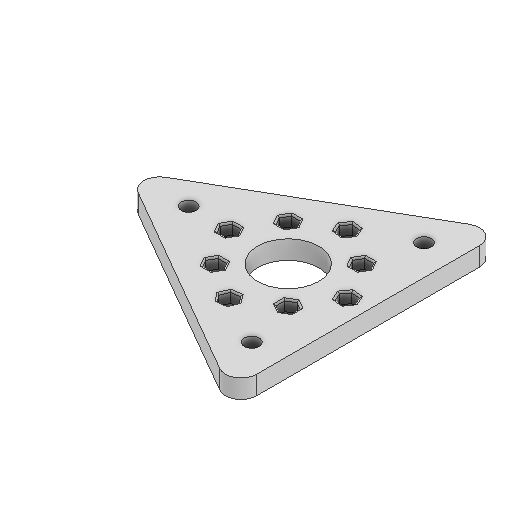
# Autodesk Inventor part: AP-1-02-planetCarrier
Saved by Autodesk Inventor 2025.1 (Build 291241020, 241B)
## iProperties
Created: 2023-07-11
Part Number: AP-1-02-planetCarrier
Material: Generic
Document SubType Name: Modeling
Designer: t205b
Density: 1 g/cm^3
Appearance: Default
Author: t205b
Autodesk Inventor part; units mm, degrees
ref_plane "YZ Plane" through (0, 0, 0) normal (1, 0, 0) x (0, 1, 0)
ref_plane "XZ Plane" through (0, 0, 0) normal (0, 1, 0) x (-1, 0, 0)
ref_plane "XY Plane" through (0, 0, 0) normal (0, 0, 1) x (1, 0, 0)
sketch "Sketch1" plane through (0, 0, 0) normal (0, 1, 0) x (-1, 0, 0)
  line L0 (153.9793, -88.9) -> (0, 0)
  line L1 (0, 0) -> (0, -177.8)
  line L2 (0, -177.8) -> (153.9793, -88.9)
  circle A0 centre (51.3264, -88.9) radius 19.65
  line L3 (76.9897, -133.35) -> (61.1514, -105.9174) construction
  line L4 (76.9897, -44.45) -> (61.1514, -71.8826) construction
  line L5 (31.6764, -88.9) -> (0, -88.9) construction
  circle A1 centre (115.2355, -88.9) radius 6.1085
  circle A2 centre (19.3719, -144.2469) radius 6.1085
  circle A3 centre (19.3719, -33.5531) radius 6.1085
  line L6 (19.3719, -144.2469) -> (51.3264, -88.9) construction
  line L7 (51.3264, -88.9) -> (115.2355, -88.9) construction
  line L8 (51.3264, -88.9) -> (19.3719, -33.5531) construction
  arc A4 (19.8862, -150.3337) -> (18.8576, -150.3337) centre (19.3719, -150.3604) ccw
  arc A5 (21.7419, -149.8769) -> (20.7637, -150.1947) centre (21.2611, -150.0612) ccw
  arc A6 (23.3657, -148.8689) -> (22.5335, -149.4735) centre (22.9653, -149.1928) ccw
  arc A7 (24.5985, -147.4086) -> (23.9939, -148.2407) centre (24.3178, -147.8403) ccw
  arc A8 (25.3197, -145.6387) -> (25.0019, -146.617) centre (25.1862, -146.1361) ccw
  arc A9 (25.4587, -143.7326) -> (25.4587, -144.7612) centre (25.4854, -144.2469) ccw
  arc A10 (25.0019, -141.8768) -> (25.3197, -142.8551) centre (25.1862, -142.3577) ccw
  arc A11 (23.9939, -140.2531) -> (24.5985, -141.0853) centre (24.3178, -140.6535) ccw
  arc A12 (22.5335, -139.0203) -> (23.3657, -139.6249) centre (22.9653, -139.301) ccw
  arc A13 (20.7637, -138.2991) -> (21.7419, -138.6169) centre (21.2611, -138.4326) ccw
  arc A14 (18.8576, -138.1601) -> (19.8862, -138.1601) centre (19.3719, -138.1334) ccw
  arc A15 (17.0018, -138.6169) -> (17.9801, -138.2991) centre (17.4827, -138.4326) ccw
  arc A16 (15.3781, -139.6249) -> (16.2102, -139.0203) centre (15.7785, -139.301) ccw
  arc A17 (14.1452, -141.0853) -> (14.7499, -140.2531) centre (14.426, -140.6535) ccw
  arc A18 (13.4241, -142.8551) -> (13.7419, -141.8768) centre (13.5576, -142.3577) ccw
  arc A19 (13.2851, -144.7612) -> (13.2851, -143.7326) centre (13.2584, -144.2469) ccw
  arc A20 (13.7419, -146.617) -> (13.4241, -145.6387) centre (13.5576, -146.1361) ccw
  arc A21 (14.7499, -148.2407) -> (14.1452, -147.4086) centre (14.426, -147.8403) ccw
  arc A22 (16.2102, -149.4735) -> (15.3781, -148.8689) centre (15.7785, -149.1928) ccw
  arc A23 (17.9801, -150.1947) -> (17.0018, -149.8769) centre (17.4827, -150.0612) ccw
  arc A24 (121.0824, -87.1314) -> (121.2963, -88.1376) centre (121.2155, -87.6289) ccw
  arc A25 (120.2497, -85.4112) -> (120.764, -86.302) centre (120.53, -85.8432) ccw
  arc A26 (118.9262, -84.0325) -> (119.6906, -84.7208) centre (119.3263, -84.3568) ccw
  arc A27 (117.2414, -83.1302) -> (118.1811, -83.5486) centre (117.7221, -83.315) ccw
  arc A28 (115.3603, -82.7928) -> (116.3833, -82.9003) centre (115.8746, -82.82) ccw
  arc A29 (113.467, -83.0531) -> (114.4731, -82.8393) centre (113.9645, -82.9201) ccw
  arc A30 (111.7467, -83.8858) -> (112.6375, -83.3715) centre (112.1788, -83.6056) ccw
  arc A31 (110.368, -85.2093) -> (111.0563, -84.4449) centre (110.6923, -84.8093) ccw
  arc A32 (109.4658, -86.8941) -> (109.8842, -85.9544) centre (109.6506, -86.4134) ccw
  arc A33 (109.1283, -88.7752) -> (109.2358, -87.7523) centre (109.1555, -88.261) ccw
  arc A34 (113.2297, -94.6698) -> (112.29, -94.2514) centre (112.749, -94.485) ccw
  arc A35 (115.1108, -95.0072) -> (114.0878, -94.8997) centre (114.5965, -94.98) ccw
  arc A36 (117.0041, -94.7469) -> (115.998, -94.9607) centre (116.5066, -94.8799) ccw
  arc A37 (118.7244, -93.9142) -> (117.8336, -94.4285) centre (118.2923, -94.1944) ccw
  arc A38 (120.1031, -92.5907) -> (119.4148, -93.3551) centre (119.7788, -92.9907) ccw
  arc A39 (121.0053, -90.9059) -> (120.5869, -91.8456) centre (120.8205, -91.3866) ccw
  arc A40 (121.3428, -89.0248) -> (121.2353, -90.0477) centre (121.3156, -89.539) ccw
  arc A41 (111.5449, -93.7675) -> (110.7805, -93.0792) centre (111.1448, -93.4432) ccw
  arc A42 (110.2214, -92.3888) -> (109.7071, -91.498) centre (109.9411, -91.9567) ccw
  arc A43 (109.3887, -90.6686) -> (109.1748, -89.6624) centre (109.2556, -90.1711) ccw
  arc A44 (14.9168, -29.3738) -> (15.6812, -28.6856) centre (15.2812, -29.0099) ccw
  arc A45 (13.8434, -30.9551) -> (14.3577, -30.0643) centre (14.0774, -30.4963) ccw
  arc A46 (13.3112, -32.7906) -> (13.525, -31.7845) centre (13.392, -32.282) ccw
  arc A47 (13.3722, -34.7008) -> (13.2647, -33.6778) centre (13.2919, -34.1921) ccw
  arc A48 (14.0205, -36.4987) -> (13.6021, -35.559) centre (13.7869, -36.0397) ccw
  arc A49 (15.1926, -38.0082) -> (14.5044, -37.2438) centre (14.8287, -37.6438) ccw
  arc A50 (16.7739, -39.0816) -> (15.8831, -38.5673) centre (16.3151, -38.8475) ccw
  arc A51 (18.6094, -39.6138) -> (17.6033, -39.4) centre (18.1008, -39.533) ccw
  arc A52 (20.5196, -39.5528) -> (19.4966, -39.6603) centre (20.0109, -39.6331) ccw
  arc A53 (22.3175, -38.9045) -> (21.3778, -39.3229) centre (21.8585, -39.138) ccw
  arc A54 (25.3716, -32.4054) -> (25.4791, -33.4283) centre (25.4519, -32.9141) ccw
  arc A55 (24.7233, -30.6075) -> (25.1416, -31.5472) centre (24.9568, -31.0665) ccw
  arc A56 (23.5511, -29.098) -> (24.2394, -29.8624) centre (23.9151, -29.4624) ccw
  arc A57 (21.9699, -28.0246) -> (22.8607, -28.5389) centre (22.4286, -28.2586) ccw
  arc A58 (20.1343, -27.4924) -> (21.1405, -27.7062) centre (20.643, -27.5732) ccw
  arc A59 (18.2241, -27.5534) -> (19.2471, -27.4459) centre (18.7328, -27.4731) ccw
  arc A60 (16.4263, -28.2017) -> (17.366, -27.7833) centre (16.8853, -27.9681) ccw
  arc A61 (25.4326, -34.3155) -> (25.2188, -35.3217) centre (25.3518, -34.8242) ccw
  arc A62 (24.9004, -36.1511) -> (24.3861, -37.0419) centre (24.6663, -36.6098) ccw
  arc A63 (23.827, -37.7323) -> (23.0625, -38.4206) centre (23.4626, -38.0963) ccw
  circle A64 centre (19.3719, -144.2469) radius 4.7879
  circle A65 centre (115.2355, -88.9) radius 4.7879
  circle A66 centre (19.3719, -33.5531) radius 4.7879
  point P0 (21.7419, -149.8769)
  point P1 (23.3657, -148.8689)
  point P2 (22.5335, -149.4735)
  point P3 (24.5985, -147.4086)
  point P4 (25.0019, -141.8768)
  point P5 (25.3197, -142.8551)
  point P6 (23.9939, -140.2531)
  point P7 (22.5335, -139.0203)
  point P8 (23.3657, -139.6249)
  point P9 (20.7637, -138.2991)
  point P10 (21.7419, -138.6169)
  point P11 (19.8862, -138.1601)
  point P12 (17.9801, -138.2991)
  point P13 (15.3781, -139.6249)
  point P14 (16.2102, -139.0203)
  point P15 (14.1452, -141.0853)
  point P16 (14.7499, -140.2531)
  point P17 (13.2851, -144.7612)
  point P18 (13.7419, -146.617)
  point P19 (13.4241, -145.6387)
  point P20 (14.7499, -148.2407)
  point P21 (14.1452, -147.4086)
  point P22 (16.2102, -149.4735)
  point P23 (15.3781, -148.8689)
  point P24 (17.0018, -149.8769)
  point P25 (15.6812, -28.6856)
  point P26 (13.8434, -30.9551)
  point P27 (14.3577, -30.0643)
  point P28 (13.3112, -32.7906)
  point P29 (13.525, -31.7845)
  point P30 (14.0205, -36.4987)
  point P31 (15.1926, -38.0082)
  point P32 (14.5044, -37.2438)
  point P33 (16.7739, -39.0816)
  point P34 (15.8831, -38.5673)
  point P35 (18.6094, -39.6138)
  point P36 (17.6033, -39.4)
  point P37 (20.5196, -39.5528)
  point P38 (19.4966, -39.6603)
  point P39 (22.3175, -38.9045)
  point P40 (21.3778, -39.3229)
  point P41 (25.3716, -32.4054)
  point P42 (25.4791, -33.4283)
  point P43 (24.7233, -30.6075)
  point P44 (25.1416, -31.5472)
  point P45 (23.5511, -29.098)
  point P46 (24.2394, -29.8624)
  point P47 (21.9699, -28.0246)
  point P48 (22.8607, -28.5389)
  point P49 (20.1343, -27.4924)
  point P50 (21.1405, -27.7062)
  point P51 (18.2241, -27.5534)
  point P52 (16.4263, -28.2017)
  point P53 (17.366, -27.7833)
  point P54 (25.2188, -35.3217)
  point P55 (24.9004, -36.1511)
  point P56 (24.3861, -37.0419)
  point P57 (23.827, -37.7323)
  point P58 (23.0625, -38.4206)
  point P59 (121.0824, -87.1314)
  point P60 (120.764, -86.302)
  point P61 (118.1811, -83.5486)
  point P62 (115.3603, -82.7928)
  point P63 (116.3833, -82.9003)
  point P64 (111.7467, -83.8858)
  point P65 (112.6375, -83.3715)
  point P66 (109.8842, -85.9544)
  point P67 (109.2358, -87.7523)
  point P68 (121.3428, -89.0248)
  point P69 (110.2214, -92.3888)
  point P70 (109.7071, -91.498)
  point P71 (109.3887, -90.6686)
  point P72 (109.1748, -89.6624)
  point P73 (113.2297, -94.6698)
  point P74 (112.29, -94.2514)
  point P75 (115.1108, -95.0072)
  point P76 (117.0041, -94.7469)
  point P77 (117.8336, -94.4285)
  point P78 (119.4148, -93.3551)
  dimension "d4" = 12.217
  dimension "d0" = 177.8
  dimension "d1" = 39.3
  dimension "d2" = 102.6529
  dimension "d3" = 63.9091
  dimension "d5" = 120
  dimension "d6" = 120
  dimension "d11" = 0.515
  dimension "d15" = 360
  dimension "d19" = 360
  dimension "d55" = 9.5758
  dimension "d56" = 63.9091
  dimension "d59" = 360
  constraints: 123 point on circle, 64 centre point, 18 end point, 6 equal length, 3 line through centre, 3 midpoint, 2 perpendicular, 1 coincident, 1 horizontal, 1 point on line, 1 vertical, 1 vertical alignment, 337 other
  measures "d0" distance of L0.end L1.end
  measures "d1" diameter of A0
  measures "d2" distance of L1.end L6.end
  measures "d3" distance of L6.start L6.end
  measures "d5" angle of L6 L7
  measures "d6" angle of L8 L7
  measures "d11" radius of A4
  measures "d55" diameter of A64
  measures "d56" distance of A64.centre L6.end
extrude "Extrusion1" add sketch "Sketch1" along normal blind 12 contours L2 L1 L0 | A1 A40 A39 A38 A37 A36 A35 A34 A41 A42 A43 A33 A32 A31 A30 A29 A28 A27 A26 A25 A24 | A24 A1 | A1 A40 | A25 A1 | A1 A39 | A26 A1 | A1 A38 | A27 A1 | A1 A37 | A28 A1 | A1 A36 | A29 A1 | A1 A35 | A30 A1 | A1 A34 | A31 A1 | A1 A41 | A32 A1 | A1 A42 | A33 A1 | A1 A43 | A2 A9 | A9 A2 A8 A7 A6 A5 A4 A23 A22 A21 A20 A19 A18 A17 A16 A15 A14 A13 A12 A11 A10 | A10 A2 | A2 A8 | A11 A2 | A2 A7 | A12 A2 | A2 A6 | A13 A2 | A2 A5 | A14 A2 | A2 A4 | A15 A2 | A2 A23 | A16 A2 | A2 A22 | A17 A2 | A2 A21 | A18 A2 | A2 A20 | A19 A2 | A3 A61 A62 A63 A53 A52 A51 A50 A49 A48 A47 A46 A45 A44 A60 A59 A58 A57 A56 A55 A54 | A54 A3 | A3 A61 | A55 A3 | A3 A62 | A56 A3 | A3 A63 | A57 A3 | A3 A53 | A58 A3 | A3 A52 | A59 A3 | A3 A51 | A60 A3 | A3 A50 | A44 A3 | A3 A49 | A45 A3 | A3 A48 | A46 A3 | A3 A47
fillet "Fillet1" radius 10 3 edges at (0, 6, -177.8) (0, 6, 0) (-153.9793, 6, -88.9)
sketch "Sketch3" plane through (0, 12, 0) normal (0, 1, 0) x (1, 0, 0)
  circle A0 centre (-27.7564, 65.33) radius 2.85
  circle A1 centre (-74.8964, 65.33) radius 2.85
  circle A2 centre (-74.8964, 112.47) radius 2.85
  circle A3 centre (-27.7564, 112.47) radius 2.85
  circle A4 centre (-51.3264, 88.9) radius 19.65 projected
  circle A5 centre (-51.3264, 126.9) radius 2.85
  circle A6 centre (-89.3264, 88.9) radius 2.85
  circle A7 centre (-51.3264, 50.9) radius 2.85
  circle A8 centre (-13.3264, 88.9) radius 2.85
  circle A9 centre (-89.3264, 88.9) radius 5
  circle A10 centre (-51.3264, 50.9) radius 5
  circle A11 centre (-74.8964, 65.33) radius 5
  circle A12 centre (-27.7564, 65.33) radius 5
  circle A13 centre (-13.3264, 88.9) radius 5
  circle A14 centre (-74.8964, 112.47) radius 5
  circle A15 centre (-51.3264, 126.9) radius 5
  circle A16 centre (-27.7564, 112.47) radius 5
  line L0 (-47.8195, 46.3137) -> (-53.5448, 45.5697)
  line L1 (-53.5448, 45.5697) -> (-57.0518, 50.156)
  line L2 (-57.0518, 50.156) -> (-54.8334, 55.4863)
  line L3 (-54.8334, 55.4863) -> (-49.108, 56.2303)
  line L4 (-49.108, 56.2303) -> (-45.6011, 51.644)
  line L5 (-45.6011, 51.644) -> (-47.8195, 46.3137)
  line L6 (-22.7179, 62.511) -> (-27.6785, 59.557)
  line L7 (-27.6785, 59.557) -> (-32.717, 62.376)
  line L8 (-32.717, 62.376) -> (-32.795, 68.149)
  line L9 (-32.795, 68.149) -> (-27.8344, 71.103)
  line L10 (-27.8344, 71.103) -> (-22.7959, 68.284)
  line L11 (-22.7959, 68.284) -> (-22.7179, 62.511)
  line L12 (-10.9778, 83.6258) -> (-16.7197, 84.2289)
  line L13 (-16.7197, 84.2289) -> (-19.0684, 89.5031)
  line L14 (-19.0684, 89.5031) -> (-15.6751, 94.1742)
  line L15 (-15.6751, 94.1742) -> (-9.9332, 93.5711)
  line L16 (-9.9332, 93.5711) -> (-7.5845, 88.2969)
  line L17 (-7.5845, 88.2969) -> (-10.9778, 83.6258)
  line L18 (-21.9829, 112.47) -> (-24.8697, 107.47)
  line L19 (-24.8697, 107.47) -> (-30.6432, 107.47)
  line L20 (-30.6432, 107.47) -> (-33.5299, 112.47)
  line L21 (-33.5299, 112.47) -> (-30.6432, 117.47)
  line L22 (-30.6432, 117.47) -> (-24.8697, 117.47)
  line L23 (-24.8697, 117.47) -> (-21.9829, 112.47)
  line L24 (-45.6011, 126.156) -> (-49.108, 121.5697)
  line L25 (-49.108, 121.5697) -> (-54.8334, 122.3137)
  line L26 (-54.8334, 122.3137) -> (-57.0518, 127.644)
  line L27 (-57.0518, 127.644) -> (-53.5448, 132.2303)
  line L28 (-53.5448, 132.2303) -> (-47.8195, 131.4863)
  line L29 (-47.8195, 131.4863) -> (-45.6011, 126.156)
  line L30 (-72.0097, 107.47) -> (-77.7832, 107.47)
  line L31 (-77.7832, 107.47) -> (-80.6699, 112.47)
  line L32 (-80.6699, 112.47) -> (-77.7832, 117.47)
  line L33 (-77.7832, 117.47) -> (-72.0097, 117.47)
  line L34 (-72.0097, 117.47) -> (-69.1229, 112.47)
  line L35 (-69.1229, 112.47) -> (-72.0097, 107.47)
  line L36 (-83.5529, 88.9) -> (-86.4397, 83.9)
  line L37 (-86.4397, 83.9) -> (-92.2132, 83.9)
  line L38 (-92.2132, 83.9) -> (-95.0999, 88.9)
  line L39 (-95.0999, 88.9) -> (-92.2132, 93.9)
  line L40 (-92.2132, 93.9) -> (-86.4397, 93.9)
  line L41 (-86.4397, 93.9) -> (-83.5529, 88.9)
  line L42 (-69.1229, 65.33) -> (-72.0097, 60.33)
  line L43 (-72.0097, 60.33) -> (-77.7832, 60.33)
  line L44 (-77.7832, 60.33) -> (-80.6699, 65.33)
  line L45 (-80.6699, 65.33) -> (-77.7832, 70.33)
  line L46 (-77.7832, 70.33) -> (-72.0097, 70.33)
  line L47 (-72.0097, 70.33) -> (-69.1229, 65.33)
  point P0 (0, 0)
  point P1 (-24.0544, 68.6978)
  point P2 (-22.9739, 66.9833)
  point P3 (-78.5985, 68.6978)
  point P4 (-79.679, 66.9833)
  point P5 (-46.7103, 48.9788)
  point P6 (-22.7569, 65.3975)
  point P7 (-9.2811, 85.9614)
  point P8 (-23.4263, 114.97)
  point P9 (-46.7103, 128.8212)
  point P10 (-70.5663, 109.97)
  point P11 (-84.9963, 91.4)
  point P12 (-70.5663, 67.83)
  point P13 (-27.7564, 117.47)
  point P14 (-23.4263, 109.97)
  point P15 (-32.0866, 114.97)
  point P16 (-32.0866, 109.97)
  point P17 (-27.7564, 107.47)
  point P18 (-51.9707, 121.9417)
  point P19 (-47.3546, 123.8629)
  point P20 (-55.9426, 124.9788)
  point P21 (-55.2983, 129.9371)
  point P22 (-50.6822, 131.8583)
  point P23 (-70.5663, 114.97)
  point P24 (-74.8964, 107.47)
  point P25 (-74.8964, 117.47)
  point P26 (-79.2266, 114.97)
  point P27 (-79.2266, 109.97)
  point P28 (-89.3264, 83.9)
  point P29 (-84.9963, 86.4)
  point P30 (-93.6566, 86.4)
  point P31 (-93.6566, 91.4)
  point P32 (-89.3264, 93.9)
  point P33 (-17.894, 86.866)
  point P34 (-13.8487, 83.9274)
  point P35 (-17.3717, 91.8386)
  point P36 (-12.8042, 93.8726)
  point P37 (-8.7589, 90.934)
  point P38 (-74.8964, 70.33)
  point P39 (-70.5663, 62.83)
  point P40 (-79.2266, 67.83)
  point P41 (-79.2266, 62.83)
  point P42 (-74.8964, 60.33)
  point P43 (-25.3151, 69.6935)
  point P44 (-25.1982, 61.034)
  point P45 (-30.3147, 69.626)
  point P46 (-32.756, 65.2625)
  point P47 (-30.1977, 60.9665)
  point P48 (-55.2983, 47.8629)
  point P49 (-50.6822, 45.9417)
  point P50 (-55.9426, 52.8212)
  point P51 (-51.9707, 55.8583)
  point P52 (-47.3546, 53.9371)
  dimension "d41" = 10
  dimension "d21" = 5.7
  dimension "d22" = 5.7
  dimension "d23" = 47.14
  dimension "d24" = 47.14
  dimension "d25" = 23.57
  dimension "d26" = 23.57
  dimension "d27" = 5.7
  dimension "d51" = 38
  dimension "d52" = 38
  dimension "d53" = 38
  dimension "d54" = 38
  constraints: 96 end point, 16 coincident, 8 centre point, 8 midpoint, 5 equal radius, 4 horizontal, 4 horizontal alignment, 4 point on line, 4 vertical alignment, 128 other
  measures "d21" diameter of A0
  measures "d22" diameter of A1
  measures "d23" distance of A2.centre A1.centre
  measures "d24" distance of A3.centre A2.centre
  measures "d25" horizontal distance of A4.centre A1.centre
  measures "d26" horizontal distance of A4.centre A1.centre
  measures "d27" diameter of A5
  measures "d51" distance of A7.centre A4.centre
  measures "d52" distance of A5.centre A4.centre
  measures "d53" distance of A8.centre A4.centre
  measures "d54" distance of A6.centre A4.centre
extrude "Extrusion2" cut sketch "Sketch3" against normal through all contours A0 | A1 | A2 | A3 | A5 | A6 | A7 | A8
extrude "Extrusion3" cut sketch "Sketch3" against normal blind 7 contours A0 | A1 | A2 | A3 | A5 | A6 | A7 | A8 | A9 | A9 L41 L36 | A9 L40 L41 | L36 L37 A9 | A9 L39 L40 | L37 L38 A9 | A9 L38 L39 | A10 | A10 L4 L5 | A10 L3 L4 | L5 L0 A10 | A10 L2 L3 | L0 L1 A10 | A10 L1 L2 | A11 | A11 L47 L42 | A11 L46 L47 | L42 L43 A11 | A11 L45 L46 | L43 L44 A11 | A11 L44 L45 | A12 | L11 L6 A12 | A12 L10 L11 | A12 L9 L10 | L6 L7 A12 | A12 L8 L9 | L7 L8 A12 | A13 | A13 L16 L17 | A13 L15 L16 | L17 L12 A13 | A13 L14 L15 | L12 L13 A13 | A13 L13 L14 | A14 | A14 L34 L35 | A14 L33 L34 | L35 L30 A14 | A14 L32 L33 | L30 L31 A14 | A14 L31 L32 | A15 | A15 L29 L24 | A15 L28 L29 | L24 L25 A15 | A15 L27 L28 | L25 L26 A15 | A15 L26 L27 | A16 | A16 L23 L18 | A16 L22 L23 | L18 L19 A16 | A16 L21 L22 | L19 L20 A16 | A16 L20 L21
fillet "Fillet2" radius 1 48 edges at (-74.8964, 12, -60.33) (-70.5663, 12, -62.83) (-70.5663, 12, -67.83) (-74.8964, 12, -70.33) (-79.2266, 12, -67.83) (-79.2266, 12, -62.83) (-55.2983, 12, -47.8629) (-50.6822, 12, -45.9417) (-46.7103, 12, -48.9788) (-47.3546, 12, -53.9371) (-51.9707, 12, -55.8583) (-55.9426, 12, -52.8212) (-25.1982, 12, -61.034) (-30.1977, 12, -60.9665) (-32.756, 12, -65.2625) (-30.3147, 12, -69.626) (-25.3151, 12, -69.6935) (-22.7569, 12, -65.3975) (-13.8487, 12, -83.9274) (-17.894, 12, -86.866) (-17.3717, 12, -91.8386) (-12.8042, 12, -93.8726) (-8.7589, 12, -90.934) (-9.2811, 12, -85.9614) (-23.4263, 12, -109.97) (-27.7564, 12, -107.47) (-32.0866, 12, -109.97) (-32.0866, 12, -114.97) (-27.7564, 12, -117.47) (-23.4263, 12, -114.97) (-55.9426, 12, -124.9788) (-55.2983, 12, -129.9371) (-50.6822, 12, -131.8583) (-46.7103, 12, -128.8212) (-47.3546, 12, -123.8629) (-51.9707, 12, -121.9417) (-70.5663, 12, -109.97) (-70.5663, 12, -114.97) (-74.8964, 12, -117.47) (-79.2266, 12, -114.97) (-79.2266, 12, -109.97) (-74.8964, 12, -107.47) (-84.9963, 12, -86.4) (-89.3264, 12, -83.9) (-93.6566, 12, -86.4) (-93.6566, 12, -91.4) (-89.3264, 12, -93.9) (-84.9963, 12, -91.4)
equation "\"d24\" = d23"
equation "\"d25\" = 0.5 * d23"
equation "\"d26\" = 0.5 * d24"
equation "\"d52\" = d51"
equation "\"d53\" = d52"
equation "\"d54\" = d52"
body "Solid1"
